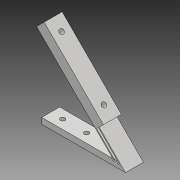
# Autodesk Inventor part: charge
Saved by Autodesk Inventor 2018 (Build 220112000, 112)
## iProperties
Created: 2017-06-02
Part Number: charge
Material: Generic
Document SubType Name: Modeling
Designer: AYUSH SHUKLA
Density: 1 g/cm^3
Appearance: Default
Author: AYUSH SHUKLA
Autodesk Inventor part; units mm, degrees
ref_plane "YZ Plane" through (0, 0, 0) normal (1, 0, 0) x (0, 1, 0)
ref_plane "XZ Plane" through (0, 0, 0) normal (0, 1, 0) x (-1, 0, 0)
ref_plane "XY Plane" through (0, 0, 0) normal (0, 0, 1) x (1, 0, 0)
sketch "Sketch1" plane through (475.3607, 0, -304.7358) normal (0, 1, 0) x (-1, 0, 0)
  line L0 (-230.3144, -553.6037) -> (1418.8804, 1095.5912)
  line L1 (1257.2358, 1257.2358) -> (0, 0)
  line L2 (0, 0) -> (143.6839, -143.6842)
  line L3 (1418.8804, 1095.5912) -> (1257.2358, 1257.2358)
  line L4 (143.684, -143.6842) -> (-233.396, -520.7642)
  line L5 (-338.0775, -553.6037) -> (107.7631, -107.763)
  line L6 (89.8025, -89.8027) -> (-468.1591, -647.7642)
  line L7 (-468.1591, -647.7642) -> (1309.841, -647.7642)
  line L8 (1309.841, -520.7642) -> (-161.5539, -520.7642)
  line L9 (-161.5539, -520.7642) -> (-212.3539, -571.5642)
  line L10 (-212.3539, -571.5642) -> (-230.3144, -553.6037)
  line L11 (-233.396, -520.7642) -> (-269.317, -520.7642)
  line L12 (-269.317, -520.7642) -> (-320.117, -571.5642)
  line L13 (-320.117, -571.5642) -> (-338.0775, -553.6037)
  line L14 (1309.841, -647.7642) -> (1309.841, -520.7642)
  line L15 (107.7631, -107.763) -> (143.684, -143.6842)
  line L16 (143.6839, -143.6842) -> (-233.396, -520.7642)
  line L17 (-233.396, -520.7642) -> (-269.317, -520.7642)
  line L18 (-269.317, -520.7642) -> (-320.117, -571.5642)
  line L19 (-320.117, -571.5642) -> (-338.0775, -553.6037)
  line L20 (-338.0775, -553.6037) -> (107.7629, -107.7632)
  constraints: 42 end point, 3 collinear, 2 point on line
extrude "Extrusion1" add sketch "Sketch1" along normal blind 381
sketch "Sketch2" plane through (943.5197, 0, -952.5) normal (0, 0, -1) x (-1, 0, 0)
  circle A0 centre (1524, 190.5) radius 50.8
  circle A1 centre (1016, 190.5) radius 50.8
  line L0 (1778, 0) -> (1778, 381) projected
  line L1 (0, 381) -> (1778, 381) projected
  point P0 (0, -381)
  dimension "d6" = 101.6
  dimension "d3" = 101.6
  dimension "d5" = 508
  dimension "d4" = 0
  dimension "d8" = 254
  dimension "d7" = 190.5
  constraints: 2 centre point
  measures "d6" diameter of A0
  measures "d3" diameter of A1
  measures "d5" distance of A0.centre A1.centre
  measures "d4" vertical distance of A1.centre A0.centre
  measures "d8" distance from line of L0 A0.centre
  measures "d7" distance from line of L1 A0.centre
extrude "Extrusion2" cut sketch "Sketch2" against normal up to surface (127 mm away)
scale "Scale1" factors (0.03937, 0.03937, 0.03937) then translate (-114.2403, 183, -32.4136) bodies 1
sketch "Sketch3" plane through (-95.5254, 183, -44.4111) normal (0.7071068, 0, 0.7071068) x (0.7071068, 0, -0.7071068)
  circle A0 centre (-59.9999, 7.5) radius 2
  circle A1 centre (-9.9999, 7.5) radius 2
  line L0 (-69.9999, 15) -> (0, 15) projected
  line L1 (-69.9999, 0) -> (-69.9999, 15) projected
  point P0 (36.1433, -183)
  dimension "d15" = 4
  dimension "d16" = 4
  dimension "d17" = 7.5
  dimension "d18" = 0
  dimension "d19" = 50
  dimension "d20" = 10
  constraints: 2 centre point
  measures "d15" diameter of A0
  measures "d16" diameter of A1
  measures "d17" distance from line of L0 A0.centre
  measures "d18" vertical distance of A1.centre A0.centre
  measures "d19" distance of A1.centre A0.centre
  measures "d20" distance from line of L1 A0.centre
extrude "Extrusion3" cut sketch "Sketch3" against normal blind 10
body "Solid1"
